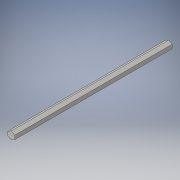
# Autodesk Inventor part: 20 in stock hex shaft
Saved by Autodesk Inventor 2016 SP2 (Build 200236200, 236)
## iProperties
Created: 2018-01-13
Part Number: 20 in stock hex shaft
Material: Generic
Document SubType Name: Modeling
Designer: CAD
Density: 1 g/cm^3
Appearance: Default
Author: CAD
Autodesk Inventor part; units mm, degrees
ref_plane "YZ Plane" through (0, 0, 0) normal (1, 0, 0) x (0, 1, 0)
ref_plane "XZ Plane" through (0, 0, 0) normal (0, 1, 0) x (-1, 0, 0)
ref_plane "XY Plane" through (0, 0, 0) normal (0, 0, 1) x (1, 0, 0)
sketch "Sketch1" plane through (0, 0, 0) normal (0, 0, 1) x (1, 0, 0)
  line L0 (10.9985, 6.35) -> (10.9985, -6.35)
  line L1 (10.9985, -6.35) -> (0, -12.7)
  line L2 (0, -12.7) -> (-10.9985, -6.35)
  line L3 (-10.9985, -6.35) -> (-10.9985, 6.35)
  line L4 (-10.9985, 6.35) -> (0, 12.7)
  line L5 (0, 12.7) -> (10.9985, 6.35)
  point P0 (0, 0)
  point P1 (0, 0)
  dimension "d0" = 12.7
  constraints: 12 end point, 1 coincident, 1 vertical, 13 other
  measures "d0" distance of L4.end L0.start
extrude "Extrusion1" add sketch "Sketch1" along normal blind 508
body "Solid1"
